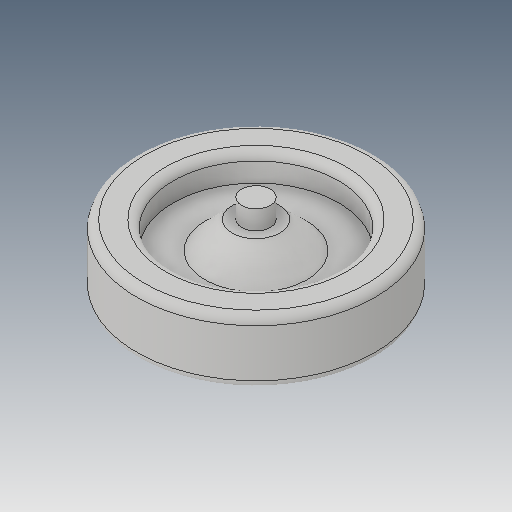
# Autodesk Inventor part: 自由輪パーツ3
Saved by Autodesk Inventor 2020.3 (Build 243373000, 373)
## iProperties
Part Number: 自由輪パーツ3
Material: 一般
Document SubType Name: Modeling
Designer: highs
Density: 1 g/cm^3
Appearance: 既定
Description: https://www.monotaro.com/p/3519/5946/
Stock Number: ナンシン プレート式 自在、ゴム(B入り)車 車輪径D 150Φmm、許容荷重 160daN、STC-150CBC
Author: highs
Autodesk Inventor part; units mm, degrees
ref_plane "YZ Plane" through (0, 0, 0) normal (1, 0, 0) x (0, 1, 0)
ref_plane "XZ Plane" through (0, 0, 0) normal (0, 1, 0) x (-1, 0, 0)
ref_plane "XY Plane" through (0, 0, 0) normal (0, 0, 1) x (1, 0, 0)
sketch "スケッチ1" plane through (0, 0, 0) normal (0, 0, 1) x (1, 0, 0)
  line L0 (0, 0) -> (0, 64)
  line L1 (0, 32) -> (75, 32) construction
  line L2 (0, 0) -> (9, 0)
  line L3 (9, 0) -> (9, 12)
  line L4 (9, 12) -> (15, 12)
  line L5 (15, 12) -> (32, 29)
  line L6 (32, 29) -> (52, 29)
  line L7 (52, 29) -> (52, 12)
  line L8 (52, 12) -> (75, 12)
  line L9 (75, 12) -> (75, 32)
  line L10 (0, 64) -> (9, 64)
  line L11 (9, 64) -> (9, 52)
  line L12 (9, 52) -> (15, 52)
  line L13 (15, 52) -> (32, 35)
  line L14 (32, 35) -> (52, 35)
  line L15 (52, 35) -> (52, 52)
  line L16 (52, 52) -> (75, 52)
  line L17 (75, 52) -> (75, 32)
  dimension "d0" = 9
  dimension "d1" = 12
  dimension "d3" = 3
  dimension "d6" = 20
  dimension "d7" = 135
  dimension "d8" = 75
  dimension "d9" = 20
  dimension "d10" = 20
  dimension "d14" = 15
  constraints: 37 end point, 7 symmetric about line, 5 perpendicular, 2 horizontal, 1 midpoint, 1 parallel, 1 vertical
  measures "d0" distance of L0.start L2.end
  measures "d1" distance of L2.end L3.end
  measures "d3" distance between parallel lines of L6 L1
  measures "d6" distance between parallel lines of L4 L1
  measures "d7" angle of L5 L4
  measures "d8" distance between parallel lines of L0 L9
  measures "d9" distance of L8.end L1.end
  measures "d10" distance of L5.end L6.end
  measures "d14" distance from line of L0 L4.end
revolve "回転1" add sketch "スケッチ1" angle 360 about axis through (0, 0, 0) along (0, 1, 0)
fillet "フィレット1" radius 5 2 edges at (-75, 12, 0) (-75, 52, 0)
fillet "フィレット2" radius 5 2 edges at (-52, 12, 0) (-52, 52, 0)
